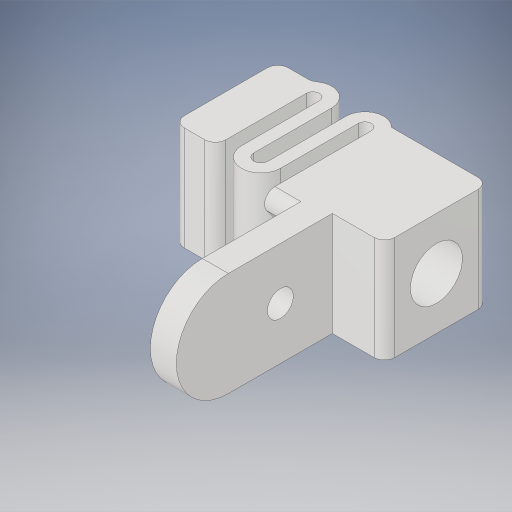
# Autodesk Inventor part: BT505_trajan20_22
Saved by Autodesk Inventor 2023 (Build 270158000, 158)
## iProperties
Company: HTBLA Kaindorf
RuleStatus: InUse
Created: 2022-11-29
Part Number: BT505_trajan20_22
Project: Zeichenmaschine_neu
Material: Kunststoff, undurchsichtig Weiß
Description: Stifthalterung_3DDruck
Document SubType Name: Modeling
Designer: trajan20
Density: 0.952 g/cm^3
Appearance: Glatt - Weiß
Mass: 13.0784 g
Surface Area: 77.7869 cm^2
Volume: 13.7378 cm^3
AfterDocNew0: iProperties-Editor_aufrufen
Author: jan
Keywords: 2022
Autodesk Inventor part; units mm, degrees
ref_plane "YZ Plane" through (0, 0, 0) normal (1, 0, 0) x (0, 1, 0)
ref_plane "XZ Plane" through (0, 0, 0) normal (0, 1, 0) x (-1, 0, 0)
ref_plane "XY Plane" through (0, 0, 0) normal (0, 0, 1) x (1, 0, 0)
sketch "Skizze3" plane through (0, 0, 0) normal (0, 0, 1) x (1, 0, 0)
  line L0 (0, 0) -> (0, 8)
  line L1 (0, 8) -> (20, 8)
  line L2 (20, 0) -> (0, 0)
  arc A0 (2.5, 21.75) -> (2.5, 16.75) centre (2.5, 19.25) ccw construction
  arc A1 (17.5, 11.75) -> (17.5, 16.75) centre (17.5, 14.25) ccw construction
  line L3 (17.5, 16.75) -> (2.5, 16.75) construction
  line L4 (2.5, 11.75) -> (17.5, 11.75) construction
  arc A2 (2.5, 11.75) -> (0.3349, 8) centre (2.5, 9.25) ccw construction
  line L5 (0, 20.5) -> (0, 40.5)
  line L6 (0, 40.5) -> (20, 40.5)
  arc A3 (0, 21.8681) -> (2.5, 15.63) centre (2.5, 19.25) ccw
  line L7 (2.5, 15.63) -> (17.5, 15.63)
  arc A4 (17.5, 12.87) -> (17.5, 15.63) centre (17.5, 14.25) ccw
  line L8 (17.5, 12.87) -> (2.5, 12.87)
  arc A5 (2.5, 12.87) -> (0, 6.6319) centre (2.5, 9.25) ccw
  arc A6 (2.5, 20.5) -> (2.5, 18) centre (2.5, 19.25) ccw
  line L9 (2.5, 18) -> (17.5, 18)
  arc A7 (17.5, 10.5) -> (17.5, 18) centre (17.5, 14.25) ccw
  line L10 (17.5, 10.5) -> (2.5, 10.5)
  arc A8 (2.5, 10.5) -> (2.5, 8) centre (2.5, 9.25) ccw
  line L11 (0, 20.5) -> (20, 20.5)
  line L12 (20, 20.5) -> (20, 20.5)
  line L13 (20, 20.5) -> (20, 30.5)
  line L14 (20, 40.5) -> (20, 30.5)
  line L15 (20, 0) -> (20, 8)
  line L16 (20, 30.5) -> (50, 30.5)
  line L17 (50, 30.5) -> (50, 25.5)
  line L18 (20, 25.5) -> (50, 25.5)
  point P0 (10, 4)
  point P1 (0, 4)
  point P2 (10, 0)
  dimension "d4" = 8
  dimension "d11" = 5
  dimension "d12" = 5
  dimension "d17" = 5
  dimension "d19" = 1.12
  dimension "d20" = 1.25
  dimension "d22" = 20
  dimension "d23" = 20
  dimension "d54" = 20
  dimension "d71" = 5
  dimension "d72" = 5
  dimension "d73" = 30
  constraints: 39 end point, 18 point on circle, 9 centre point, 9 tangent, 8 point on line, 5 perpendicular, 4 horizontal, 4 midpoint, 2 parallel, 2 vertical, 1 collinear, 1 horizontal alignment, 1 vertical alignment, 8 other
  measures "d4" distance between parallel lines of L2 L1
  measures "d11" diameter of A1
  measures "d12" diameter of A0
  measures "d17" diameter of A2
  measures "d19" distance between parallel lines of L4 L8
  measures "d20" distance between parallel lines of L4 L10
  measures "d22" distance between parallel lines of L6 L11
  measures "d23" distance between parallel lines of L5 L13
  measures "d54" distance between parallel lines of L0 L15
  measures "d71" distance between parallel lines of L11 L18
  measures "d72" distance between parallel lines of L16 L18
  measures "d73" distance between parallel lines of L17 L13
extrude "Extrusion3" add sketch "Skizze3" along normal blind 20
sketch "Skizze4" plane through (20, 30.5, 0) normal (0, 1, 0) x (1, 0, 0)
  circle A0 centre (20, -10) radius 2
  circle A1 centre (10, -10) radius 2.5
  circle A2 centre (20, -10) radius 10
  line L0 (30, 0) -> (0, 0) projected
  line L1 (0, 0) -> (0, -20) projected
  line L2 (30, -20) -> (0, -20) projected
  line L3 (30, 0) -> (30, -20) projected
  circle A3 centre (10, -10) radius 10
  line L4 (0, 0) -> (0, -20) projected
  point P0 (0, -18)
  point P1 (25, -18)
  point P2 (29, -10)
  point P3 (29.681, -7.4944)
  point P4 (-20, -18)
  point P5 (10.3125, -7.5196)
  point P6 (10.3125, -12.4804)
  point P7 (30, -10)
  point P8 (20, 0)
  point P9 (20, -20)
  point P10 (0, -10)
  point P11 (10, 0)
  point P12 (10, -20)
  dimension "d36" = 5
  dimension "d75" = 10
  dimension "d76" = 4
  constraints: 3 centre point, 3 tangent, 2 horizontal, 2 horizontal alignment, 1 coincident, 1 vertical, 3 other
  measures "d36" diameter of A1
  measures "d75" distance of A0.centre A1.centre
  measures "d76" diameter of A0
sketch "Skizze6" plane through (0, 40.5, 0) normal (0, 1, 0) x (1, 0, 0)
  circle A0 centre (10, -10) radius 5
  line L0 (20, -20) -> (0, -20) projected
  line L1 (0, 0) -> (0, -20) projected
  point P0 (10, -20)
  point P1 (0, -10)
  dimension "d51" = 10
  constraints: 2 midpoint, 1 centre point, 1 horizontal alignment, 1 vertical alignment
  measures "d51" diameter of A0
extrude "Extrusion9" cut sketch "Skizze6" against normal through all
extrude "Extrusion6" cut sketch "Skizze4" against normal through all contours L0 L3 A2 | A2 A1 | A1 A2 | A2 L3 L2
extrude "Extrusion7" add sketch "Skizze4" against normal blind 10 contours A0 A3 | A3 A0 | A3 L1 L0 | L2 L1 A3
hole "Bohrung1" at (10, 4, 0) direction (0, 0, 1) diameter 2.459 end up to face face through (10, 40.5, 10) facing (0, -1, 0) round with radius 5 far side no thread size "M3x0.5" class "6H" standard "ISO Metric profile"
fillet "Rundung3" radius 2 8 edges at (0, 40.5, 10) (20, 40.5, 10) (20, 0, 10) (20, 8, 10) (0, 0, 10) (0, 6.6319, 10) (30, 23, 0) (30, 23, 20)
equation "\"d12\" = d11"
